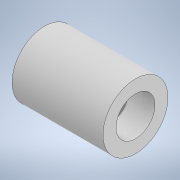
# Autodesk Inventor part: 零件2
Saved by Autodesk Inventor 2020 (Build 240168000, 168)
## iProperties
Created: 2020-12-28
Part Number: 零件2
Material: 一般
Document SubType Name: Modeling
Designer: User
Density: 1 g/cm^3
Appearance: 預設
Author: User
Autodesk Inventor part; units mm, degrees
ref_plane "YZ Plane" through (0, 0, 0) normal (1, 0, 0) x (0, 1, 0)
ref_plane "XZ Plane" through (0, 0, 0) normal (0, 1, 0) x (-1, 0, 0)
ref_plane "XY Plane" through (0, 0, 0) normal (0, 0, 1) x (1, 0, 0)
sketch "草圖1" plane through (0, 0, 0) normal (0, 0, 1) x (1, 0, 0)
  line L0 (0, 0) -> (0, 1270)
  line L1 (0, 1270) -> (3556, 1270)
  line L2 (3556, 1270) -> (3556, 0)
  line L3 (3556, 0) -> (0, 0)
  line L4 (3556, 0) -> (3556, 762)
  line L5 (3556, 762) -> (2540, 762)
  line L6 (2540, 762) -> (2540, 254)
  line L7 (2540, 254) -> (508, 254)
  line L8 (508, 254) -> (508, 0)
  dimension "d0" = 1270
  dimension "d1" = 3556
  dimension "d2" = 762
  dimension "d3" = 1016
  dimension "d4" = 508
  dimension "d5" = 2032
  constraints: 18 end point, 7 perpendicular, 2 point on line, 1 vertical
  measures "d0" distance of L0.start L0.end
  measures "d1" distance of L0.end L1.end
  measures "d2" distance of L2.end L4.end
  measures "d3" distance of L4.end L5.end
  measures "d4" distance of L5.end L6.end
  measures "d5" distance of L6.end L7.end
revolve "迴轉1" add sketch "草圖1" angle 360 about axis through (3556, 0, 0) along (-1, 0, 0) contours L0 L1 L2 L5 L6 L7 L8 L3
